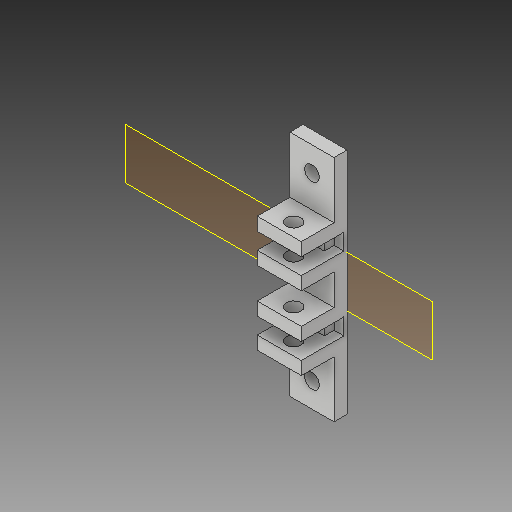
# Autodesk Inventor part: enclenchement
Saved by Autodesk Inventor 2017 (Build 210142000, 142)
## iProperties
Part Number: enclenchement
Material: Générique
Document SubType Name: Modeling
Designer: Thomas
Density: 1 g/cm^3
Appearance: Par défaut
Author: Thomas
Autodesk Inventor part; units mm, degrees
ref_plane "YZ Plane" through (0, 0, 0) normal (1, 0, 0) x (0, 1, 0)
ref_plane "XZ Plane" through (0, 0, 0) normal (0, 1, 0) x (-1, 0, 0)
ref_plane "XY Plane" through (0, 0, 0) normal (0, 0, 1) x (1, 0, 0)
ref_plane "Plan de construction1" through (24.857, 8.2218, -15) normal (0, 0, 1) x (0, 1, 0)
sketch "Esquisse1" plane through (24.857, 8.2218, -15) normal (0, 0, 1) x (0, 1, 0)
  circle A0 centre (-27.625, -11.5983) radius 2.25 projected
  circle A1 centre (27.2798, -11.5983) radius 2.25 projected
  circle A2 centre (-14.9765, -0.1949) radius 2.15 projected
  circle A3 centre (15.0235, -0.1949) radius 2.15 projected
  line L0 (34.7798, -18.3341) -> (-35.125, -18.3341) projected
  line L1 (34.7798, -4.8625) -> (34.7798, -18.3341) projected
  line L2 (20.0235, -4.8625) -> (34.7798, -4.8625) projected
  line L3 (20.0235, -4.8625) -> (20.0235, 5.1375) projected
  line L4 (20.0235, 5.1375) -> (11.0235, 5.1375) projected
  line L5 (11.0235, 5.1375) -> (11.0235, -13.773) projected
  line L6 (11.0235, -13.773) -> (-11.125, -13.773) projected
  line L7 (-11.125, -13.773) -> (-11.125, 5.1375) projected
  line L8 (-11.125, 5.1375) -> (-20.125, 5.1375) projected
  line L9 (-20.125, 5.1375) -> (-20.125, -4.8625) projected
  line L10 (-35.125, -4.8625) -> (-20.125, -4.8625) projected
  line L11 (-35.125, -18.3341) -> (-35.125, -4.8625) projected
  line L12 (34.7798, -18.3341) -> (-35.125, -18.3341)
  line L13 (-35.125, -18.3341) -> (-35.125, -4.8625)
  line L14 (-35.125, -4.8625) -> (34.7798, -4.8625)
  line L15 (34.7798, -4.8625) -> (34.7798, -18.3341)
  point P0 (-8.2218, 24.857)
  constraints: 8 end point, 2 parallel, 1 horizontal, 1 perpendicular
extrude "Extrusion1" add sketch "Esquisse1" along normal blind 4 contours L0 L11 L10 L14 L7 L6 L5 L2 L1 | L5 L6 L7 L14
sketch "Esquisse2" plane through (24.857, 8.2218, -11) normal (0, 0, 1) x (1, 0, 0)
  circle A0 centre (11.5983, -27.625) radius 2.25 projected
  circle A1 centre (11.5983, 27.2798) radius 2.25 projected
  circle A2 centre (0.1949, -14.9765) radius 2.15 projected
  circle A3 centre (0.1949, 15.0235) radius 2.15 projected
  line L0 (18.3341, 34.7798) -> (18.3341, -35.125) projected
  line L1 (4.8625, 34.7798) -> (18.3341, 34.7798) projected
  line L2 (4.8625, 20.0235) -> (4.8625, 34.7798) projected
  line L3 (4.8625, 20.0235) -> (-5.1375, 20.0235) projected
  line L4 (-5.1375, 20.0235) -> (-5.1375, 11.0235) projected
  line L5 (-5.1375, 11.0235) -> (13.773, 11.0235) projected
  line L6 (13.773, 11.0235) -> (13.773, -11.125) projected
  line L7 (13.773, -11.125) -> (-5.1375, -11.125) projected
  line L8 (-5.1375, -11.125) -> (-5.1375, -20.125) projected
  line L9 (-5.1375, -20.125) -> (4.8625, -20.125) projected
  line L10 (4.8625, -35.125) -> (4.8625, -20.125) projected
  line L11 (18.3341, -35.125) -> (4.8625, -35.125) projected
  line L12 (18.3341, -35.125) -> (18.3341, 34.7798) projected
  line L13 (4.8625, 34.7798) -> (4.8625, -35.125) projected
  line L14 (18.3341, 17.5433) -> (4.8625, 17.5433)
  line L15 (4.8625, 17.5433) -> (4.8625, 13.5433)
  line L16 (4.8625, 13.5433) -> (18.3341, 13.5433)
  line L17 (18.3341, 13.5433) -> (18.3341, 17.5433)
  line L18 (18.3341, -0.1726) -> (4.8625, -0.1726) construction
  line L19 (18.3341, 13.5433) -> (18.3341, 8.5433) construction
  line L20 (18.3341, 8.5433) -> (4.8625, 8.5433)
  line L21 (4.8625, 8.5433) -> (4.8625, 4.5433)
  line L22 (4.8625, 4.5433) -> (18.3341, 4.5433)
  line L23 (18.3341, 4.5433) -> (18.3341, 8.5433)
  line L24 (4.8625, -35.125) -> (4.8625, 34.7798)
  line L25 (18.3341, -17.8886) -> (4.8625, -17.8886)
  line L26 (4.8625, -17.8886) -> (4.8625, -13.8886)
  line L27 (4.8625, -13.8886) -> (18.3341, -13.8886)
  line L28 (18.3341, -13.8886) -> (18.3341, -17.8886)
  line L29 (18.3341, -8.8886) -> (4.8625, -8.8886)
  line L30 (4.8625, -8.8886) -> (4.8625, -4.8886)
  line L31 (4.8625, -4.8886) -> (18.3341, -4.8886)
  line L32 (18.3341, -4.8886) -> (18.3341, -8.8886)
  point P0 (-24.857, -8.2218)
  dimension "d2" = 4
  dimension "d3" = 5
  dimension "d4" = 4
  constraints: 38 end point, 10 symmetric about line, 6 point on line, 4 parallel, 2 horizontal, 2 midpoint, 2 perpendicular
  measures "d2" distance of L15.end L14.end
  measures "d3" distance of L16.end L19.end
  measures "d4" distance of L21.end L20.end
extrude "Extrusion2" add sketch "Esquisse2" along normal blind 10 contours L0 L16 L13 L14 | L0 L22 L6 L20 | L6 L22 L13 L20 | L0 L29 L6 L31 | L6 L29 L13 L31 | L0 L25 L13 L27
sketch "Esquisse3" plane through (29.7194, 25.7651, -11) normal (0, 1, 0) x (1, 0, 0)
  circle A0 centre (7.1312, -6) radius 2.25
  line L0 (13.4716, -10) -> (0, -10) projected
  point P0 (-29.7194, -11)
  dimension "d7" = 4.5
  dimension "d8" = 4
  constraints: 1 centre point
  measures "d7" diameter of A0
  measures "d8" distance from line of A0.centre L0
extrude "Extrusion3" cut sketch "Esquisse3" against normal blind 55.75
sketch "Esquisse4" plane through (24.857, 8.2218, -11) normal (0, 0, 1) x (1, 0, 0)
  line L0 (18.3341, 13.5433) -> (4.8625, 13.5433) projected
  line L1 (4.8625, 13.5433) -> (4.8625, 8.5433) projected
  line L2 (4.8625, 8.5433) -> (18.3341, 8.5433) projected
  line L3 (18.3341, 8.5433) -> (18.3341, 13.5433) projected
  line L4 (18.3341, -8.8886) -> (4.8625, -8.8886) projected
  line L5 (4.8625, -8.8886) -> (4.8625, -13.8886) projected
  line L6 (4.8625, -13.8886) -> (18.3341, -13.8886) projected
  line L7 (18.3341, -13.8886) -> (18.3341, -8.8886) projected
  line L8 (4.8625, 13.5433) -> (18.3341, 13.5433) projected
  line L9 (18.3341, 8.5433) -> (15.3341, 8.5433)
  line L10 (15.3341, 8.5433) -> (15.3341, 13.5433)
  line L11 (15.3341, 13.5433) -> (18.3341, 13.5433)
  line L12 (18.3341, 13.5433) -> (18.3341, 8.5433)
  line L13 (18.3341, -13.8886) -> (15.3341, -13.8886)
  line L14 (15.3341, -13.8886) -> (15.3341, -8.8886)
  line L15 (15.3341, -8.8886) -> (18.3341, -8.8886)
  line L16 (18.3341, -8.8886) -> (18.3341, -13.8886)
  point P0 (-24.857, -8.2218)
  dimension "d11" = 3
  dimension "d12" = 3
  constraints: 16 end point, 4 parallel, 2 horizontal, 2 perpendicular, 2 point on line
  measures "d11" distance of L10.end L11.end
  measures "d12" distance of L14.end L15.end
extrude "Extrusion4" cut sketch "Esquisse4" against normal blind 3 contours L3 L2 L10 L0 | L7 L6 L14 L4
